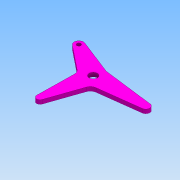
# Autodesk Inventor part: Pancake_Switch Lever 2
Saved by Autodesk Inventor 2018.1 (Build 221171000, 171)
## iProperties
Created: 2019-02-11
Part Number: Pancake_Switch Lever 2
Material: Nylon 6/6
Document SubType Name: Modeling
Designer: James
Density: 1.13 g/cm^3
Appearance: Magenta
Author: James
Autodesk Inventor part; units mm, degrees
ref_plane "YZ Plane" through (0, 0, 0) normal (1, 0, 0) x (0, 1, 0)
ref_plane "XZ Plane" through (0, 0, 0) normal (0, 1, 0) x (-1, 0, 0)
ref_plane "XY Plane" through (0, 0, 0) normal (0, 0, 1) x (1, 0, 0)
sketch "Sketch1" plane through (0, 0, 0) normal (0, 0, 1) x (1, 0, 0)
  circle A0 centre (0, 0) radius 8
  line L0 (1, 7.9373) -> (40.375, 2.9765)
  line L1 (1, -7.9373) -> (40.375, -2.9765)
  line L2 (0, 0) -> (40, 0) construction
  circle A1 centre (40, 0) radius 3
  circle A2 centre (-6.0777, -34.4683) radius 2.5
  line L3 (-3.7145, -35.2839) -> (7.5623, -2.61)
  line L4 (-8.5773, -34.4264) -> (-7.9989, 0.1339)
  line L5 (0, 0) -> (-6.0777, -34.4683) construction
  circle A3 centre (-25.9808, 15) radius 3.5
  line L6 (-24.7052, 18.2593) -> (2.9155, 7.4498)
  line L7 (-4.994, -6.2498) -> (-28.1656, 12.2657)
  line L8 (-25.9808, 15) -> (0, 0) construction
  point P0 (-3.8416, -33.3502)
  dimension "d0" = 16
  dimension "d1" = 6
  dimension "d2" = 40
  dimension "d3" = 5
  dimension "d4" = 35
  dimension "d5" = 100
  dimension "d32" = 18.082
  dimension "d36" = 30
  dimension "d37" = 7
  dimension "d38" = 150
  constraints: 18 end point, 13 point on circle, 12 tangent, 4 centre point, 2 coincident, 1 horizontal
  measures "d0" diameter of A0
  measures "d1" diameter of A1
  measures "d2" distance of L2.end point (0, 0)
  measures "d3" diameter of A2
  measures "d4" distance of L2.start L5.end
  measures "d5" angle of L2 L5
  measures "d32" angle of L3 L4
  measures "d36" distance of point (0, 0) L8.start
  measures "d37" diameter of A3
  measures "d38" angle of L2 L8
extrude "Extrusion1" add sketch "Sketch1" along normal blind 3
fillet "Fillet1" radius 5 3 edges at (5.9384, -7.3151, 1.5) (1.9881, 7.8128, 1.5) (-8.0647, -3.7962, 1.5)
sketch "Sketch2" plane through (0, 0, 3) normal (0, 0, 1) x (1, 0, 0)
  point P0 (0, 0)
  point P1 (0, 0)
  constraints: 1 coincident
hole "Hole1" at (0, 0, 3) direction (0, 0, -1) diameter 6.2 end through all
sketch "Sketch3" plane through (0, 0, 3) normal (0, 0, 1) x (1, 0, 0)
  line L0 (-8.1058, -6.2524) -> (-8.5773, -34.4264) projected
  line L1 (-3.7145, -35.2839) -> (4.9235, -10.2558) projected
  point P0 (0, 0)
  point P1 (-3.473, -19.6962)
  point P2 (-7.4498, 2.9155)
  point P3 (-8.5773, -34.4264)
  point P4 (-9.2276, -1.6271)
  dimension "d33" = 20
  dimension "d34" = 4.8571
  dimension "d35" = 4.8571
  constraints: 1 other
  measures "d33" distance of point (0, 0) point (-3.473, -19.696)
  measures "d35" distance from line of L1 point (-3.473, -19.696)
hole "Hole2" [suppressed]
sketch "Sketch4" plane through (0, 0, 3) normal (0, 0, 1) x (1, 0, 0)
  arc A0 (-8.5773, -34.4264) -> (-3.7145, -35.2839) centre (-6.0777, -34.4683) ccw projected
  arc A1 (-24.7052, 18.2593) -> (-28.1656, 12.2657) centre (-25.9808, 15) ccw projected
  point P0 (0, 0)
  constraints: 1 coincident
hole "Hole3" at (-25.9808, 15, 3) direction (0, 0, -1) diameter 3 end through all
equation "\"d34\" = d35"
body "Solid1"
